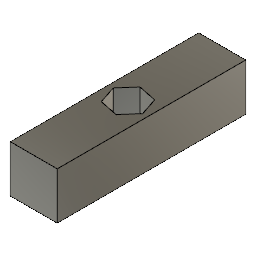
Polygon Side Print v0 (Autodesk Fusion 360 design; units mm, degrees)
Autodesk Fusion 360 part; units mm, degrees
sketch "Sketch1" plane through (0, 0, 0) normal (0, 0, 1) x (1, 0, 0)
  line L0 (0, 0) -> (10, 0)
  line L1 (10, 0) -> (10, -40)
  line L2 (10, -40) -> (0, -40)
  line L3 (0, -40) -> (0, 0)
  dimension "d1" = 40
  dimension "d2" = 10
  constraint horizontal L0
  constraint vertical L1
  constraint horizontal L2
  constraint vertical L3
  constraint coincident L0.start L3.end
  measures "d1" distance of L0.start L2.end
  measures "d2" distance of L0.start L0.end
extrude "Extrude1" add sketch "Sketch1" along normal blind 10
sketch "Sketch2" plane through (0, 0, 10) normal (0, 0, 1) x (-1, 0, 0)
  line L0 (0, 40) -> (-10, 40)
  line L1 (-10, 40) -> (-10, 0)
  line L2 (-10, 0) -> (0, 0)
  line L3 (0, 0) -> (0, 40)
  line L4 (-6.2649, 23.7947) -> (-8.9188, 20.8019)
  line L5 (-8.9188, 20.8019) -> (-7.6539, 17.0072)
  line L6 (-7.6539, 17.0072) -> (-3.7351, 16.2053)
  line L7 (-3.7351, 16.2053) -> (-1.0812, 19.1981)
  line L8 (-1.0812, 19.1981) -> (-2.3461, 22.9928)
  line L9 (-2.3461, 22.9928) -> (-6.2649, 23.7947)
  point P0 (-5, 20)
  dimension "d5" = 4
  measures "d5" distance of L4.start P0
extrude "Extrude2" cut sketch "Sketch2" against normal blind 5 contours L4 L5 L6 L7 L8 L9
